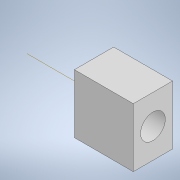
# Autodesk Inventor part: Angle Bracket
Saved by Autodesk Inventor 2022 (Build 260153000, 153)
## iProperties
Created: 2022-04-03
Part Number: Angle Bracket
Material: Generic
Document SubType Name: Modeling
Designer: Nick
Density: 1 g/cm^3
Appearance: Default
Author: Nick
Autodesk Inventor part; units mm, degrees
ref_plane "YZ Plane" through (0, 0, 0) normal (1, 0, 0) x (0, 1, 0)
ref_plane "XZ Plane" through (0, 0, 0) normal (0, 1, 0) x (-1, 0, 0)
ref_plane "XY Plane" through (0, 0, 0) normal (0, 0, 1) x (1, 0, 0)
sketch "Sketch1" plane through (0, 0, 0) normal (0, 0, 1) x (1, 0, 0)
  line L0 (0, 0) -> (0, 9.525)
  line L1 (0, 9.525) -> (9.525, 9.525)
  line L2 (9.525, 9.525) -> (9.525, 8.525)
  line L3 (9.525, 8.525) -> (1, 8.525)
  line L4 (1, 8.525) -> (1, 0)
  line L5 (1, 0) -> (0, 0)
  dimension "d0" = 9.525
  dimension "d1" = 9.525
  dimension "d2" = 1
  constraints: 12 end point, 2 horizontal, 2 perpendicular, 2 vertical, 1 parallel
  measures "d0" distance of L0.start L0.end
  measures "d1" distance of L0.end L1.end
  measures "d2" distance of L1.end L2.end
extrude "Extrusion1" add sketch "Sketch1" along normal blind 6.35
sketch "Sketch2" plane through (0, 0, 0) normal (-1, 0, 0) x (0, 0, 1)
  line L0 (6.35, 9.525) -> (6.35, 0) projected
  line L1 (0, 9.525) -> (6.35, 9.525) projected
  point P0 (0, 0)
  point P1 (3.175, 4.7625)
  point P2 (6.35, 4.7625)
  point P3 (3.175, 9.525)
  constraints: 2 midpoint, 1 horizontal alignment, 1 vertical alignment
sketch "Sketch4" plane through (0, 0, 6.35) normal (0, 0, 1) x (1, 0, 0)
  line L0 (0, 0) -> (1, 0) projected
  line L1 (9.525, 8.525) -> (9.525, 9.525) projected
  line L2 (0, 0) -> (9.525, 0)
  line L3 (9.525, 0) -> (9.525, 9.525)
  line L4 (9.525, 9.525) -> (0, 9.525)
  line L5 (0, 9.525) -> (0, 0)
  constraints: 8 end point, 2 parallel, 1 horizontal, 1 perpendicular
extrude "Extrusion2" add sketch "Sketch4" against normal up to surface (6.35 mm away)
sketch "Sketch3" plane through (0, 0, 0) normal (-1, 0, 0) x (0, 0, 1)
  line L0 (6.35, 9.525) -> (6.35, 0) projected
  line L1 (0, 9.525) -> (6.35, 9.525) projected
  point P0 (0, 0)
  point P1 (3.175, 4.7625)
  point P2 (6.35, 4.7625)
  point P3 (3.175, 9.525)
  constraints: 2 midpoint, 1 horizontal alignment, 1 vertical alignment
hole "Hole1" at (0, 4.7625, 3.175) direction (1, 0, 0) diameter 4 end through all
equation "\"d1\" = d0"
body "Solid1"
